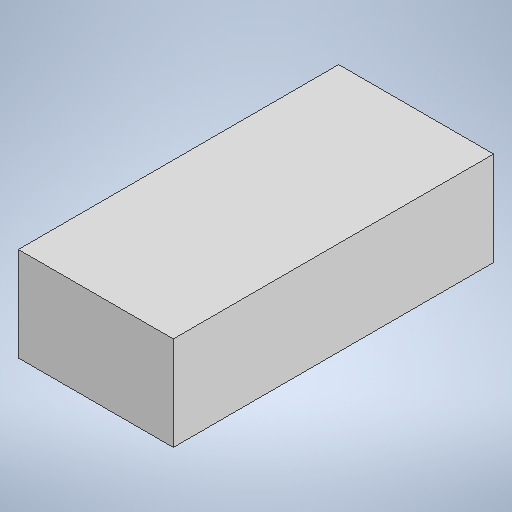
# Autodesk Inventor part: USB_HUB_MOUNT
Saved by Autodesk Inventor 2025.1 (Build 291241000, 241)
## iProperties
Created: 2024-10-18
Part Number: USB_HUB_MOUNT
Material: Generic
Document SubType Name: Modeling
Designer: shubh
Density: 1 g/cm^3
Appearance: Default
Author: shubh
Autodesk Inventor part; units mm, degrees
ref_plane "YZ Plane" through (0, 0, 0) normal (1, 0, 0) x (0, 1, 0)
ref_plane "XZ Plane" through (0, 0, 0) normal (0, 1, 0) x (-1, 0, 0)
ref_plane "XY Plane" through (0, 0, 0) normal (0, 0, 1) x (1, 0, 0)
sketch "Sketch1" plane through (0, 0, 0) normal (0, 0, 1) x (1, 0, 0)
  line L0 (-21.0034, 11.156) -> (-8.7163, 11.156)
  line L1 (-8.7163, 11.156) -> (-8.7163, 3.7039)
  line L2 (-8.7163, 3.7039) -> (-21.0034, 3.7039)
  line L3 (-21.0034, 3.7039) -> (-21.0034, 11.156)
  point P0 (0, 0)
  constraints: 8 end point, 2 parallel, 1 horizontal, 1 perpendicular
extrude "Extrusion1" add sketch "Sketch1" along normal blind 25.4
body "Solid1"
